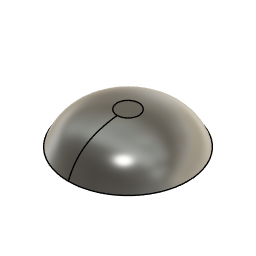
hub_roof_2 (Autodesk Fusion 360 design; units mm, degrees)
Autodesk Fusion 360 part; units mm, degrees
note: some values were not read from the file. Set by a fixed rule: which sketch regions a step uses.
sketch "Sketch1" plane through (0, 0, 0) normal (1, 0, 0) x (0, 1, 0)
  spline S0 degree 5 poles (-20, 0) (-22.7257, -0.3253) (-28.0984, -1.0502) (-35.9212, -2.3607) (-45.8716, -4.5618) (-57.453, -8.1224) (-68.0948, -12.571) (-77.709, -17.9907) (-86.2289, -24.4443) (-93.6692, -31.9182) (-100.0996, -40.3463) (-104.4963, -47.7952) (-107.3992, -53.7549) (-109.1618, -57.8911) (-110, -60) knots 0 0 0 0 0 0 0.1 0.2 0.3 0.4 0.5 0.6 0.7 0.8 0.9 1 1 1 1 1 1
  spline S1 degree 3 poles (-19.6445, -2.9789) (-34.008, -4.693) (-47.0407, -7.6194) (-58.39, -11.9827) (-67.6436, -15.5402) (-75.7205, -20.0828) (-82.5658, -25.7517) (-91.5958, -33.2299) (-98.5876, -42.6658) (-103.9793, -53.7643) (-105.1319, -56.1368) (-106.2094, -58.5851) (-107.2121, -61.108) knots 0 0 0 0 0.320426 0.320426 0.320426 0.581685 0.581685 0.581685 0.926327 0.926327 0.926327 1 1 1 1
  line L0 (0, 0) -> (0, -2.9702)
  line L1 (-110, -60) -> (-106.765, -60)
  line L2 (-20, 0) -> (0, 0)
  line L3 (-19.6445, -2.9789) -> (0, -2.9702)
  point P0 (-80, -20)
  dimension "d1" = 110
  dimension "d2" = 60
  dimension "d3" = 80
  dimension "d4" = 20
  dimension "d5" = -3
  dimension "d18" = 20
  constraint vertical L0
  constraint coincident S1 L1.end
  constraint perpendicular L0 L1
  constraint coincident L0.start L2.end
  constraint perpendicular L0 L2
  measures "d1" distance of L0.start S0.end
  measures "d2" distance of L0.start S0.end
  measures "d3" horizontal distance of L0.start P0
  measures "d4" vertical distance of L0.start P0
  measures "d18" distance of L0.start S0.start
revolve "Revolve1" add sketch "Sketch1" angle 360 about axis through (0, 0, 1.75) along (0, 0, 1)
ref_plane "WorkPlane1" through (0, 0, -2) normal (0, 0, 1) x (1, 0, 0)
sketch "Sketch2" plane through (0, 0, -2) normal (0, 0, 1) x (1, 0, 0)
  circle A0 centre (0, 0) radius 22.5
  dimension "d7" = 45
  constraint coincident A0.centre origin
  measures "d7" diameter of A0
extrude "Extrude1" add sketch "Sketch2" against normal blind 25
sketch "Sketch3" plane through (0, 0, -27) normal (0, 0, -1) x (1, 0, 0)
  circle A0 centre (0, 0) radius 22.5
  circle A1 centre (10.6066, -10.6066) radius 2.05
  circle A2 centre (3.8823, 14.4889) radius 2.05
  circle A3 centre (-14.4889, -3.8823) radius 2.05
  line L0 (0, 0) -> (10.6066, -10.6066) construction
  dimension "d10" = 4.1
  dimension "d14" = 360
  dimension "d19" = 15
  constraint coincident A0.centre L0.start
  constraint coincident A1.centre L0.end
  measures "d10" diameter of A1
  measures "d19" distance of A0.centre A1.centre
extrude "Extrude2" cut sketch "Sketch3" against normal blind 15 contours A1 | A2 | A3
sketch "Sketch4" plane through (0, 0, -27) normal (0, 0, -1) x (1, 0, 0)
  circle A0 centre (10.6066, -10.6066) radius 2.05
  circle A1 centre (-14.4889, -3.8823) radius 2.05
  circle A2 centre (3.8823, 14.4889) radius 2.05
  circle A3 centre (0, 0) radius 22.5
  circle A4 centre (0, 0) radius 5
  dimension "d20" = 10
  constraint concentric A3 A4
  measures "d20" diameter of A4
extrude "Extrude3" cut sketch "Sketch4" against normal blind 5 contours A4
